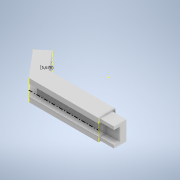
# Autodesk Inventor part: LAMPA1
Saved by Autodesk Inventor 2020 (Build 240168000, 168)
## iProperties
Created: 2019-11-22
Part Number: LAMPA1
Material: Všeobecné
Document SubType Name: Modeling
Designer: kotel
Density: 1 g/cm^3
Appearance: Výchozí
Author: kotel
Autodesk Inventor part; units mm, degrees
ref_plane "YZ Plane" through (0, 0, 0) normal (1, 0, 0) x (0, 1, 0)
ref_plane "XZ Plane" through (0, 0, 0) normal (0, 1, 0) x (-1, 0, 0)
ref_plane "XY Plane" through (0, 0, 0) normal (0, 0, 1) x (1, 0, 0)
sketch "Náčrt1" plane through (0, 0, 0) normal (0, 1, 0) x (-1, 0, 0)
  line L0 (0, 0) -> (50, 0)
  line L1 (50, 0) -> (66.0697, -19.1511)
  line L2 (50, 0) -> (75, 0) construction
  line L3 (66.0697, -19.1511) -> (58.4092, -25.579)
  line L4 (0, -12) -> (0, 0)
  line L5 (58.6554, -25.3724) -> (47.4347, -12)
  line L6 (47.4347, -12) -> (0, -12)
  dimension "d0" = 50
  dimension "d2" = 25
  dimension "d3" = 50
  dimension "d4" = 10
  dimension "d5" = 12
  constraints: 14 end point, 3 horizontal, 2 perpendicular, 1 equal length, 1 parallel, 1 point on line
  measures "d0" distance of L0.start L0.end
  measures "d2" distance of L0.end L1.end
  measures "d3" angle of L1 L2
  measures "d4" distance of L1.end L3.end
  measures "d5" distance of L4.start L0.start
extrude "Vysunutí1" add sketch "Náčrt1" along normal blind 15
sketch "Náčrt8" plane through (-66.0697, 0, -19.1511) normal (-0.6428, 0, -0.766) x (-0.766, 0, 0.6428)
  line L0 (-9.6786, 0) -> (-9.6786, 15) projected
  line L1 (-9.6786, 7.5) -> (0, 7.5)
  line L2 (0, 0) -> (0, 15) projected
  point P0 (-38.3022, 0)
  constraints: 2 end point, 2 midpoint
sketch "Náčrt9" plane through (-50, 0, 0) normal (-0.766, 0, 0.6428) x (0.6428, 0, 0.766)
  line L0 (-25, 0) -> (-25, 15) projected
  line L1 (0, 0) -> (0, 15) projected
sketch "Náčrt10" plane through (-50, 0, 0) normal (0, 0, 1) x (1, 0, 0)
  line L0 (0, 0) -> (0, 15) projected
  line L1 (0, 7.5) -> (50, 7.5)
  line L2 (50, 0) -> (50, 15) projected
  constraints: 2 end point, 2 midpoint
sketch "Náčrt11" plane through (0, 0, 0) normal (1, 0, 0) x (0, 0, -1)
  line L0 (0, 0) -> (0, 15) projected
  line L1 (0, 7.5) -> (12, 7.5)
  line L2 (12, 0) -> (12, 15) projected
  line L3 (0, 3.5) -> (4, 3.5)
  line L4 (4, 3.5) -> (4, 11.5)
  line L5 (4, 11.5) -> (0, 11.5)
  line L6 (0, 11.5) -> (0, 3.5)
  point P0 (0, 7.5)
  point P1 (0, 11.5)
  dimension "d64" = 4
  dimension "d65" = 8
  constraints: 10 end point, 3 midpoint, 2 parallel, 1 horizontal, 1 perpendicular, 1 point on line, 1 other
  measures "d64" distance of L5.end L4.end
  measures "d65" distance of L4.end L3.end
extrude "Vysunutí10" cut sketch "Náčrt11" against normal through all
sketch "Náčrt21" plane through (-66.0697, 0, -19.1511) normal (-0.6428, 0, -0.766) x (-0.766, 0, 0.6428)
  line L0 (0, 0) -> (0, 15) projected
  line L1 (0, 3.5) -> (-4, 3.5)
  line L2 (-4, 3.5) -> (-4, 11.5)
  line L3 (-4, 11.5) -> (0, 11.5)
  line L4 (0, 11.5) -> (0, 3.5)
  point P0 (-38.3022, 0)
  point P1 (0, 7.5)
  point P2 (0, 11.5)
  dimension "d68" = 4
  dimension "d69" = 8
  constraints: 8 end point, 3 perpendicular, 2 parallel, 1 horizontal, 1 midpoint, 1 point on line, 1 other
  measures "d68" distance of L2.end L3.end
  measures "d69" distance of L1.end L2.end
extrude "Vysunutí11" cut sketch "Náčrt21" against normal through all
sketch "Náčrt22" plane through (-63.0055, 3.5, -21.7223) normal (-0.766, 0, 0.6428) x (0.6428, 0, 0.766)
  line L0 (0, -3.5) -> (0, 11.5) projected
  line L1 (0, 4) -> (23.1348, 4)
  line L2 (23.1348, 8) -> (23.1348, 0) projected
  circle A0 centre (7.71, 4) radius 2.8
  point P0 (57.1394, -3.5)
  dimension "d72" = 5.6
  constraints: 2 end point, 2 midpoint, 1 centre point, 1 point on line, 1 other
  measures "d72" diameter of A0
sketch "Náčrt25" plane through (-58.6554, 0, -25.3724) normal (-0.6428, 0, -0.766) x (-0.766, 0, 0.6428)
  line L0 (5.6786, 3.5) -> (5.6786, 11.5) projected
  line L1 (5.6786, 5.4735) -> (0, 5.4735)
  line L2 (0, 0) -> (0, 15) projected
  point P0 (-28.6236, 0)
  dimension "d73" = 5.6786
  constraints: 2 end point, 2 point on line, 1 horizontal
  measures "d73" distance of L1.start L1.end
extrude "Vysunutí12" cut sketch "Náčrt22" against normal blind 2
sketch "Náčrt27" plane through (-56.5175, 7.5, -17.1016) normal (-0.766, 0, 0.6428) x (0.6428, 0, 0.766)
  circle A0 centre (0, 0) radius 2.8 projected
  line L0 (0, -2.8) -> (0, 2.8)
  line L1 (-2.7895, 0) -> (2.8105, 0)
  circle A1 centre (0, 0) radius 2.45
  point P0 (49.4294, -7.5)
  dimension "d79" = 5.6
  dimension "d80" = 4.9
  constraints: 4 end point, 2 point on circle, 1 centre point, 1 coincident, 1 horizontal, 1 midpoint, 1 perpendicular, 1 vertical, 1 other
  measures "d79" distance of L1.start L1.end
  measures "d80" diameter of A1
extrude "Vysunutí14" cut sketch "Náčrt27" against normal through all contours A1 L0 L1 | L1 L0 A1 | L0 L1 A1 | A1 L1 L0
sketch "Náčrt28" plane through (0, 0, 0) normal (1, 0, 0) x (0, 0, -1)
  line L0 (0, 0) -> (0, 3.5) projected
  line L1 (12, 0) -> (12, 15) projected
  line L2 (0, 0) -> (12, 0) projected
  line L3 (0, 15) -> (12, 15) projected
  line L4 (0, 11.5) -> (0, 15) projected
  line L5 (1, 0.6751) -> (10, 0.6751)
  line L6 (4, 11.5) -> (4, 3.5) projected
  line L7 (1, 2.8249) -> (5, 2.8249)
  line L8 (1, 12.1751) -> (5, 12.1751)
  line L9 (1, 14.3249) -> (10, 14.3249)
  line L10 (5, 2.8249) -> (5, 12.1751)
  line L11 (9.8978, 0.6751) -> (9.8978, 14.3249)
  line L12 (1, 0.6751) -> (1, 2.8249)
  line L13 (1, 12.1751) -> (1, 14.3249)
  line L14 (4, 7.5) -> (12, 7.5)
  point P0 (5, 7.5)
  point P1 (9.8978, 7.5)
  point P2 (5.5, 0.6751)
  point P3 (5.5, 14.3249)
  point P4 (1, 13.25)
  point P5 (0, 13.25)
  point P6 (1, 1.75)
  point P7 (0, 1.75)
  constraints: 18 end point, 10 midpoint, 3 horizontal alignment, 2 parallel, 2 perpendicular, 2 point on line, 2 vertical, 1 collinear, 1 horizontal, 1 vertical alignment, 5 other
extrude "Vysunutí15" add sketch "Náčrt28" along normal blind 10
